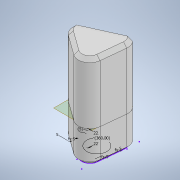
# Autodesk Inventor part: body
Saved by Autodesk Inventor 2020 (Build 240168000, 168)
## iProperties
Created: 2019-07-02
Part Number: body
Material: Generic
Document SubType Name: Modeling
Designer: erwin
Density: 1 g/cm^3
Appearance: Default
case_thickness: 2.500 mm
Author: erwin
Autodesk Inventor part; units mm, degrees
ref_plane "YZ Plane" through (0, 0, 0) normal (1, 0, 0) x (0, 1, 0)
ref_plane "XZ Plane" through (0, 0, 0) normal (0, 1, 0) x (-1, 0, 0)
ref_plane "XY Plane" through (0, 0, 0) normal (0, 0, 1) x (1, 0, 0)
sketch "Sketch1" plane through (0, 0, 0) normal (0, 1, 0) x (-1, 0, 0)
  line L0 (24.2988, -12.4688) -> (-6.8086, -26.4489)
  line L1 (-22.9477, -14.8089) -> (-19.5011, 19.1209)
  line L2 (-1.3511, 27.2777) -> (26.3097, 7.328)
  line L3 (22.2492, 9.0918) -> (5.2492, 9.0918)
  line L4 (5.2492, 9.0918) -> (5.2492, -12.9082)
  line L5 (5.2492, -12.9082) -> (22.2492, -12.9082)
  line L6 (27.2492, -7.9082) -> (27.2492, 4.0918)
  arc A0 (27.2492, 4.0918) -> (22.2492, 9.0918) centre (22.2492, 4.0918) ccw
  arc A1 (22.2492, -12.9082) -> (27.2492, -7.9082) centre (22.2492, -7.9082) ccw
  line L7 (-18.9983, 14.7224) -> (-10.4983, 0)
  line L8 (-10.4983, 0) -> (8.5542, 11)
  line L9 (8.5542, 11) -> (0.0542, 25.7224)
  line L10 (-6.7759, 27.5526) -> (-17.1682, 21.5526)
  arc A2 (-17.1682, 21.5526) -> (-18.9983, 14.7224) centre (-14.6682, 17.2224) ccw
  arc A3 (0.0542, 25.7224) -> (-6.7759, 27.5526) centre (-4.2759, 23.2224) ccw
  line L11 (-3.2508, -23.8142) -> (5.2492, -9.0918)
  line L12 (5.2492, -9.0918) -> (-13.8034, 1.9082)
  line L13 (-13.8034, 1.9082) -> (-22.3034, -12.8142)
  line L14 (-20.4733, -19.6444) -> (-10.081, -25.6444)
  arc A4 (-10.081, -25.6444) -> (-3.2508, -23.8142) centre (-7.581, -21.3142) ccw
  arc A5 (-22.3034, -12.8142) -> (-20.4733, -19.6444) centre (-17.9733, -15.3142) ccw
  arc A6 (24.2988, -12.4688) -> (26.3097, 7.328) centre (19.5894, -1.9899) ccw
  arc A7 (-1.3511, 27.2777) -> (-19.5011, 19.1209) centre (-8.0714, 17.9599) ccw
  arc A8 (-22.9477, -14.8089) -> (-6.8086, -26.4489) centre (-11.518, -15.97) ccw
  point P0 (0, 0)
  point P1 (0, 0)
  point P2 (42.4488, -4.3119)
  point P3 (-24.9586, -34.6057)
  point P4 (-17.4901, 38.9177)
  point P5 (27.2492, -12.9082)
  point P6 (-2.4458, 30.0526)
  point P7 (-24.8034, -17.1444)
  dimension "d0" = 22
  dimension "d1" = 22
  dimension "d2" = 5
  dimension "d5" = 360
  dimension "d8" = 5
  dimension "d9" = 5
  dimension "d10" = 5
  dimension "d11" = 5
  constraints: 30 end point, 18 point on circle, 13 point on line, 12 tangent, 9 centre point, 3 equal radius, 2 parallel, 1 coincident, 1 horizontal, 1 perpendicular, 53 other
  measures "d0" distance of point (27.249, -12.908) L4.end
  measures "d1" distance of L4.end L3.end
  measures "d2" radius of A0
  measures "d8" distance from line of L0 A1.centre
  measures "d9" distance from line of L1 A5.centre
  measures "d10" distance from line of L1 A2.centre
  measures "d11" distance from line of L2 A0.centre
extrude "Extrusion1" add sketch "Sketch1" along normal blind 130
thicken "Thicken1" operation add thickness 4.5 both sides no extend neighbours yes toward (0.9948803, 0, 0.1010599) faces at (20.6499, 43.3333, 7.8109) (15.4184, 86.6667, 26.792) (-17.0894, 43.3333, 13.9779) (19.908, 86.6667, -23.8181) (-3.5605, 43.3333, -21.7888) (-27.9121, 86.6667, -9.9094)
chamfer "Chamfer1" distance 5 angle 45 12 edges at (-10.5897, 130, -23.5634) (-35.496, 130, -3.6057) (-15.1116, 130, 20.9526) (14.6254, 130, 32.5433) (25.7013, 130, 2.6107) (20.8706, 130, -28.9376) (-10.5897, 0, -23.5634) (-35.496, 0, -3.6057) (-15.1116, 0, 20.9526) (14.6254, 0, 32.5433) (25.7013, 0, 2.6107) (20.8706, 0, -28.9376)
shell "Shell1" thickness 2.5 removed faces 0
ref_plane "Work Plane2" through (0, 45, 0) normal (0, -1, 0) x (1, 0, 0)
split body "Split1" result two bodies by plane through (0, 45, 0) normal (0, -1, 0) first body at (-0.6411, 0.5, 6.3117)
sketch "Sketch3" plane through (-23.6693, 127.5, -11.0682) normal (0, -1, 0) x (0.9121216, 0, -0.4099197)
  line L0 (8.5374, 25.9392) -> (17.5557, 5.8725) projected
  line L1 (26.628, 24.1015) -> (4.7406, 26.3249) projected
  line L2 (15.9913, 9.3535) -> (28.8604, 27.1968) projected
  point P0 (17.0522, 19.7981)
extrude "Extrusion2" add sketch "Sketch3" along normal blind 20 bodies 3
fillet "Fillet1" radius 3 6 edges at (-5.2492, 107.5, 0) (2.6246, 107.5, -4.5459) (2.6246, 107.5, 4.5459) (-5.2492, 127.5, 0) (2.6246, 127.5, -4.5459) (2.6246, 127.5, 4.5459)
thicken "Thicken2" operation add thickness 4 both sides no extend neighbours yes toward (0.5, 0, -0.8660254) bodies 3 faces at (5.2492, 115.1667, -3.0306) (-5.2492, 119.8333, 3.0306) (0, 115.1667, 6.0612)
equation "\"d9\" = d8"
equation "\"d10\" = d8"
equation "\"d11\" = d8"
equation "\"d20\" = case_thickness"
equation "\"case_thickness\" = 2.5"
equation "\"case_thickness_extra\" = 2"
body "Solid2"
body "Solid3"
